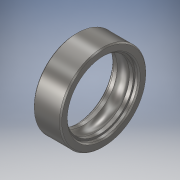
# Autodesk Inventor part: Bearings - Outer Race
Saved by Autodesk Inventor 2019 (Build 230136000, 136)
## iProperties
Created: 2020-12-03
Part Number: Bearings - Outer Race
Material: Stainless Steel
Document SubType Name: Modeling
Designer: Anass Hamdi
Density: 8 g/cm^3
Appearance: Semi-Polished
Author: Anass Hamdi
Autodesk Inventor part; units mm, degrees
ref_plane "YZ Plane" through (0, 0, 0) normal (1, 0, 0) x (0, 1, 0)
ref_plane "XZ Plane" through (0, 0, 0) normal (0, 1, 0) x (-1, 0, 0)
ref_plane "XY Plane" through (0, 0, 0) normal (0, 0, 1) x (1, 0, 0)
sketch "Sketch1" plane through (0, 0, 0) normal (0, 0, 1) x (1, 0, 0)
  line L0 (3.5, -8.5) -> (2.5, -8.5) construction
  line L1 (-2.5, -8.5) -> (-3.5, -8.5) construction
  line L2 (-2.5, -8.5) -> (-2.5, -9)
  line L3 (2.5, -8.5) -> (2.5, -9)
  line L4 (-2.5, -9) -> (-3.5, -9)
  line L5 (-3.5, -9) -> (-3.5, -11)
  line L6 (2.5, -9) -> (3.5, -9)
  line L7 (3.5, -9) -> (3.5, -11)
  line L8 (3.5, -11) -> (-3.5, -11)
  line L9 (-4.9, 0) -> (4.9, 0) projected
  line L10 (0, -8.5) -> (0, -7.25) construction
  arc A0 (-1.5612, -8.5) -> (1.5612, -8.5) centre (0, -7.25) ccw
  line L11 (2.5, -8.5) -> (1.5612, -8.5)
  line L12 (-1.5612, -8.5) -> (-2.5, -8.5)
  line L13 (1.5612, -8.5) -> (-1.5612, -8.5) construction
  point P0 (0, 0)
  dimension "d1" = 7
  dimension "d2" = 1
  dimension "d3" = 1
  dimension "d4" = 0.5
  dimension "d5" = 2
  dimension "d19" = 1.25
  dimension "d20" = 4
  constraints: 26 end point, 7 horizontal, 3 perpendicular, 3 vertical, 2 point on circle, 1 centre point, 1 coincident
  measures "d1" distance of L0.start L1.end
  measures "d2" distance of L0.end L0.start
  measures "d3" distance of L1.start L1.end
  measures "d4" distance of L1.start L2.end
  measures "d5" distance of L4.end L5.end
  measures "d19" distance of L10.start L10.end
  measures "d20" diameter of A0
revolve "Revolution1" add sketch "Sketch1" angle 360 about axis through (-10, 0, 0) along (1, 0, 0)
chamfer "Chamfer1" distance 0.3 angle 45 4 edges at (3.5, 9, 0) (-3.5, 11, 0) (-3.5, 9, 0) (3.5, 11, 0)
body "Solid1"
